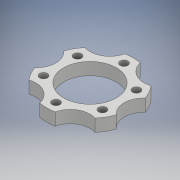
# Autodesk Inventor part: Spacer8mm
Saved by Autodesk Inventor 2018 (Build 220112000, 112)
## iProperties
Created: 2018-01-22
Part Number: Spacer8mm
Material: Generic
Document SubType Name: Modeling
Designer: eroldan
Density: 1 g/cm^3
Appearance: Default
Author: eroldan
Autodesk Inventor part; units mm, degrees
ref_plane "YZ Plane" through (0, 0, 0) normal (1, 0, 0) x (0, 1, 0)
ref_plane "XZ Plane" through (0, 0, 0) normal (0, 1, 0) x (-1, 0, 0)
ref_plane "XY Plane" through (0, 0, 0) normal (0, 0, 1) x (1, 0, 0)
sketch "Sketch1" plane through (0, 0, 0) normal (0, 0, 1) x (1, 0, 0)
  circle A0 centre (0, 0) radius 28
  circle A1 centre (0, 0) radius 17
  point P0 (0, 22)
  dimension "d0" = 22
  dimension "d1" = 34
  dimension "d20" = 56
  constraints: 2 centre point, 2 coincident
  measures "d0" distance of point (0, 0) point (0, 22)
  measures "d1" diameter of A1
  measures "d20" diameter of A0
extrude "Extrusion1" add sketch "Sketch1" along normal mid plane 8
sketch "Sketch2" plane through (0, 0, 4) normal (0, 0, 1) x (1, 0, 0)
  point P0 (0, 0)
  point P1 (0, 22)
  dimension "d4" = 22
  measures "d4" distance of point (0, 0) point (0, 22)
hole "Hole1" at (0, 22, 4) direction (0, 0, -1) diameter 5 end through all
pattern_circular "Circular Pattern1" count 6 over 360 about axis through (0, 0, -10) along (0, 0, 1) of "Hole1"
sketch "Sketch3" plane through (0, 0, 4) normal (0, 0, 1) x (1, 0, 0)
  circle A0 centre (0, 22) radius 2.5 projected
  circle A1 centre (19.0526, 11) radius 2.5 projected
  line L0 (0, 22) -> (19.0526, 11) construction
  circle A2 centre (17.4522, 30.2282) radius 12.7296
  line L1 (9.5263, 16.5) -> (19.9795, 34.6056) construction
  point P0 (0, 0)
  constraints: 4 end point, 1 centre point, 1 midpoint, 1 perpendicular, 1 point on line
extrude "Extrusion2" cut sketch "Sketch3" against normal blind 8 contours A2
pattern_circular "Circular Pattern2" count 6 over 360 about axis through (0, 0, -10) along (0, 0, 1) of "Extrusion2"
body "Solid1"
